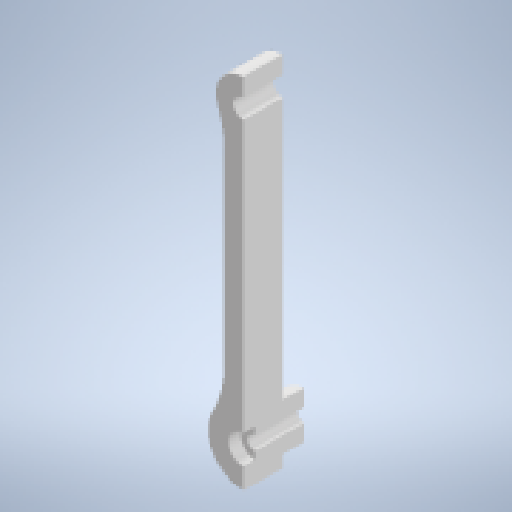
# Autodesk Inventor part: alternativeJoint
Saved by Autodesk Inventor 2025.1 (Build 291241000, 241)
## iProperties
Created: 2024-11-06
Part Number: alternativeJoint
Material: Generisch
Document SubType Name: Modeling
Designer: ZOMBULLI
Density: 1 g/cm^3
Appearance: Vorgabe
Author: ZOMBULLI
Autodesk Inventor part; units mm, degrees
ref_plane "YZ Plane" through (0, 0, 0) normal (1, 0, 0) x (0, 1, 0)
ref_plane "XZ Plane" through (0, 0, 0) normal (0, 1, 0) x (-1, 0, 0)
ref_plane "XY Plane" through (0, 0, 0) normal (0, 0, 1) x (1, 0, 0)
sketch "Skizze1" plane through (0, 0, 0) normal (0, 1, 0) x (-1, 0, 0)
  line L0 (0, 100) -> (0, 100)
  line L1 (-5, 63.8645) -> (-5, 16)
  line L2 (5, 16) -> (5, 63.8645)
  arc A0 (-7.9412, 4.2353) -> (7.9412, 4.2353) centre (0, 0) ccw
  arc A1 (5, 16) -> (7.9412, 4.2353) centre (30, 16) ccw
  arc A2 (-7.9412, 4.2353) -> (-5, 16) centre (-30, 16) ccw
  line L3 (0, -30.8) -> (0, 121.8) projected
  circle A3 centre (0, 75) radius 2.5
  arc A4 (6.5625, 72.5641) -> (-6.5625, 72.5641) centre (0, 75) ccw
  arc A5 (-5, 63.8645) -> (-6.5625, 72.5641) centre (-30, 63.8645) ccw
  arc A6 (6.5625, 72.5641) -> (5, 63.8645) centre (30, 63.8645) ccw
  point P0 (0, 0)
  point P1 (-5, 7.4833)
  point P2 (5, 7.4833)
  point P3 (-5, 70.101)
  point P4 (5, 70.101)
  dimension "d2" = 18
  dimension "d4" = 25
  dimension "d10" = 0
  dimension "d33" = 5
  dimension "d34" = 5
  dimension "d49" = 75
  dimension "d51" = 5
  dimension "d54" = 14
  constraints: 16 point on circle, 8 tangent, 7 centre point, 6 end point, 5 point on line, 3 equal radius, 1 coincident, 1 horizontal, 1 parallel, 1 perpendicular
  measures "d2" diameter of A0
  measures "d4" radius of A1
  measures "d10" distance of A0.centre point (0, 0)
  measures "d33" distance between parallel lines of L3 L1
  measures "d34" distance between parallel lines of L2 L3
  measures "d49" distance of point (0, 0) A3.centre
  measures "d51" diameter of A3
  measures "d54" diameter of A4
extrude "Extrusion1" add sketch "Skizze1" along normal blind 10
sketch "Skizze8" plane through (0, 10, 0) normal (0, 1, 0) x (1, 0, 0)
  circle A0 centre (0, 0) radius 6
  dimension "d36" = 12
  constraints: 1 centre point, 1 coincident
  measures "d36" diameter of A0
extrude "Extrusion5" add sketch "Skizze8" along normal blind 5.5
fillet "Rundung3" radius 0.2 1 edges at (-6, 15.5, 0)
fillet "Rundung4" radius 0.2 10 edges at (-5.7464, 10, 9.9366) (-5, 10, 39.9322) (5, 10, 39.9322) (5.7464, 10, 9.9366) (0, 10, -9) (-5.7464, 0, 9.9366) (-5, 0, 39.9322) (5, 0, 39.9322) (5.7464, 0, 9.9366) (0, 0, -9)
sketch "Skizze10" plane through (0, 0, 0) normal (0, -1, 0) x (1, 0, 0)
  circle A0 centre (0, 0) radius 3.65
  dimension "d41" = 7.3
  constraints: 1 centre point, 1 coincident
  measures "d41" diameter of A0
extrude "Extrusion6" cut sketch "Skizze10" against normal blind 3
sketch "Skizze11" plane through (0, 3, 0) normal (0, -1, 0) x (1, 0, 0)
  circle A0 centre (0, 0) radius 1.75
  dimension "d44" = 3.5
  constraints: 1 centre point, 1 coincident
  measures "d44" diameter of A0
extrude "Extrusion7" cut sketch "Skizze11" against normal up to next
fillet "Rundung5" radius 0.2 2 edges at (-1.75, 3, 0) (-3.65, 0, 0)
fillet "Rundung6" radius 0.2 1 edges at (-1.75, 15.5, 0)
extrude "Extrusion8" cut sketch "Skizze1" along normal up to next contours A3 L3 | L3 A3
sketch "Skizze12" plane through (0, 15.5, 0) normal (0, 1, 0) x (1, 0, 0)
  line L0 (0, -83.6989) -> (25.2084, -83.6989)
  line L1 (25.2084, -83.6989) -> (25.2084, 12.8308)
  line L2 (25.2084, 12.8308) -> (0, 12.8308)
  line L3 (0, 12.8308) -> (0, -83.6989)
  point P0 (0, 0)
  constraints: 8 end point, 2 parallel, 1 horizontal, 1 perpendicular
extrude "Extrusion9" cut sketch "Skizze12" against normal up to next
